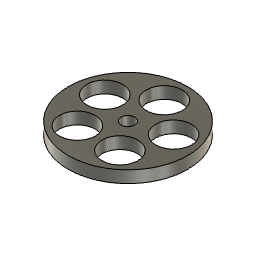
rotation_indicator (Autodesk Fusion 360 design; units mm, degrees)
Autodesk Fusion 360 part; units mm, degrees
sketch "Sketch1" plane through (0, 0, 0) normal (0, 0, 1) x (1, 0, 0)
  circle A0 centre (0, 0) radius 1.15
  circle A1 centre (0, 0) radius 10
  circle A2 centre (0.008, 6.0716) radius 3
  circle A3 centre (-5.772, 1.8838) radius 3
  circle A4 centre (-3.5753, -4.9074) radius 3
  circle A5 centre (3.5623, -4.9168) radius 3
  circle A6 centre (5.7769, 1.8686) radius 3
  dimension "d1" = 2.3
  dimension "d2" = 20
  dimension "d3" = 6
  dimension "d5" = 360
  constraint coincident A0.centre A1.centre
  measures "d1" diameter of A0
  measures "d2" diameter of A1
  measures "d3" diameter of A2
extrude "Extrude1" add sketch "Sketch1" along normal blind 2
